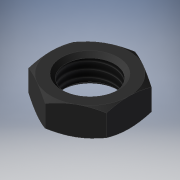
# Autodesk Inventor part: C-AC0806-nut_n
Saved by Autodesk Inventor 2019 (Build 230136000, 136)
## iProperties
Created: 2023-10-14
Part Number: C-AC0806-nut_n
Material: Generic
Catalog Web Link: www.cadenas.de
Description: C-AC_____nut-C-AC_____nut
Vendor: MISUMI
Document SubType Name: Modeling
Designer: psAdmin
Manufacturer: MISUMI
Mass: 0.259253 g
Surface Area: 3.5092 cm^2
Volume: 0.259253 cm^3
Density: 1 g/cm^3
Appearance: PSOLRGB-175-175-175
Category: PARTsolutions
Company: MISUMI
Title: C-AC0806-nut
Author: Cadenas PARTsolutions
Comments: C-AC_____nut
PSOL_IDENT_0: {$CADENAS_DATA/23d-libs/misumi/metric/29_springs/c_ac____/c_ac_____nut.prj},173 {VTYP=3D},{NB=C-AC08
PSOL_IDENT_1: 06-nut_n},{LINA=C-AC0806-nut},{NN=C-AC_____nut},{DATE=28.09.2022 00:58:34},{GEOMDATE=19.05.2022 01:1
PSOL_IDENT_2: 7:18},{VERSION=},{LINEID=200},{WBVAR=},{WBNUMERIC=}  {NB=C-AC0806-nut_n},{LINA=C-AC0806-nut},{KT=DUM
PSOL_IDENT_3: MY},{PN=C-AC0806-nut},{TYPE=C-AC0806-nut},{NO=0806},{M=8},{PITCH=1.00},{H=11.0},{I=4.0}
NB: C-AC0806-nut_n
NN: C-AC_____nut
NT: C-AC_____nut
NBSYN: $PN._n
LINA: C-AC0806-nut
CATALOG: Misumi
PN: C-AC0806-nut
NO: 0806
M: 8
PITCH: 1
H: 11
I: 4
SUPPLIER: MISUMI
ARTICLENO: C-AC0806-nut_n
BOMINFO: C-AC0806-nut
CREATOR: CADENAS GmbH
Autodesk Inventor part; units mm, degrees
sketch "Sketch_1" plane through (0, 0, 0) normal (0, 0, 1) x (1, 0, 0)
  line L0 (0, 0) -> (0, 4)
  line L1 (3.4585, 3.4585) -> (3.4585, 0.5415)
  line L2 (3.4585, 0.5415) -> (4, 0)
  line L3 (4, 0) -> (5.5, 0)
  line L4 (5.5, 0) -> (8.9641, 2)
  line L5 (8.9641, 2) -> (5.5, 4)
  line L6 (5.5, 4) -> (4, 4)
  line L7 (4, 4) -> (3.4585, 3.4585)
  constraints: 16 end point
revolve "Revolution1" add sketch "Sketch_1" angle 360 about axis through (0, 0, 0) along (0, -1, 0)
thread "Thread1" size "M8x1" class "6H" standard "ISO Metric profile" full length
sketch "Sketch_2" plane through (0, 0, 0) normal (0, 1, 0) x (1, 0, 0)
  line L0 (-50, -50) -> (50, -50)
  line L1 (50, -50) -> (50, 50)
  line L2 (50, 50) -> (-50, 50)
  line L3 (-50, 50) -> (-50, -50)
  line L4 (-5.5, -3.1754) -> (0, -6.3509)
  line L5 (0, -6.3509) -> (5.5, -3.1754)
  line L6 (5.5, -3.1754) -> (5.5, 3.1754)
  line L7 (5.5, 3.1754) -> (0, 6.3509)
  line L8 (0, 6.3509) -> (-5.5, 3.1754)
  line L9 (-5.5, 3.1754) -> (-5.5, -3.1754)
  constraints: 20 end point
extrude "Extrusion1" cut sketch "Sketch_2" along normal blind 50
ref_plane "to_body1_XY" through (0, 0, 0) normal (0, 1, 0) x (1, 0, 0)
ref_plane "to_body1_YZ" through (0, 0, 0) normal (1, 0, 0) x (0, 0, -1)
ref_plane "to_body1_ZX" through (0, 0, 0) normal (0, 0, -1) x (0, 1, 0)
ref_plane "to_body2_XY" through (0, 0, 0) normal (0, 1, 0) x (1, 0, 0)
ref_plane "to_body2_YZ" through (0, 0, 0) normal (1, 0, 0) x (0, 0, -1)
ref_plane "to_body2_ZX" through (0, 0, 0) normal (0, 0, -1) x (0, 1, 0)
body "Solid1"
